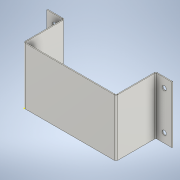
# Autodesk Inventor part: Base Valvula
Saved by Autodesk Inventor 2021 (Build 250183000, 183)
## iProperties
Created: 2021-06-01
Part Number: Base Valvula
Material: Steel AISI 1006 85 HR
Document SubType Name: Chapa
Designer: Admin
Density: 7.872 g/cm^3
Sheet Metal Rule: Default_mm
Appearance: Steel
Flat Pattern Width: 5 cm
Flat Pattern Length: 17.7756 cm
Flat Pattern Area: 88.8782 cm^2
Sheet Metal Width: 50,000 mm
Sheet Metal Length: 177,756 mm
Sheet Metal Area: 8887,816 mm^2
Mass: 52.9731 g
Surface Area: 180.926 cm^2
Volume: 6.72931 cm^3
Author: Admin
Autodesk Inventor part; units mm, degrees
ref_plane "YZ Plane" through (0, 0, 0) normal (1, 0, 0) x (0, 1, 0)
ref_plane "XZ Plane" through (0, 0, 0) normal (0, 1, 0) x (-1, 0, 0)
ref_plane "XY Plane" through (0, 0, 0) normal (0, 0, 1) x (1, 0, 0)
sketch "Boceto1" plane through (0, 0, 0) normal (0, 0, 1) x (1, 0, 0)
  line L0 (0, 0) -> (80, 0)
  line L1 (80, 0) -> (80, 50)
  line L2 (80, 50) -> (0, 50)
  line L3 (0, 50) -> (0, 0)
  dimension "d0" = 80
  dimension "d1" = 50
  measures "d0" distance of L2.end L1.end
  measures "d1" distance of L1.end L0.end
extrude "Placa1" add sketch "Boceto1" along normal blind 0.76
sketch "Boceto2" plane through (80, 50, 0) normal (1, 0, 0) x (0, 1, 0)
  line L0 (-50, 0) -> (0, 0)
  line L1 (0, 0) -> (0, 34.24)
  line L2 (0, 34.24) -> (-50, 34.24)
  line L3 (-50, 34.24) -> (-50, 0)
  constraints: 6 end point, 1 horizontal, 1 perpendicular, 1 vertical
edge flange "Pestaña1" height 35 angle 90 thickness 0.76 bend radius 0.76 thickness toward (1, 0, 0) relief tear relief width 0.76 relief depth 0.38 corner gap 0.76 corner form 0 edges at (80, 25, 0.76) (0, 25, 0.76) wall of the first edge with corners at (80, 0, 0) (80, 50, 0) (80, 50, -34.24) (80, 0, -34.24)
bend "Doblez1"
corner "Esquina1"
sketch "Boceto3" plane through (-0.76, 50, -34.24) normal (0, 0, -1) x (1, 0, 0)
  line L0 (0, -50) -> (0, 0)
  line L1 (0, 0) -> (-14.24, 0)
  line L2 (-14.24, 0) -> (-14.24, -50)
  line L3 (-14.24, -50) -> (0, -50)
  constraints: 6 end point, 1 horizontal, 1 perpendicular, 1 vertical
edge flange "Pestaña2" height 15 angle 90 thickness 0.76 bend radius 0.76 thickness toward (0, 0, -1) relief tear relief width 0.76 relief depth 0.38 corner gap 0.76 corner form 0 edges at (0, 25, -34.24) (80, 25, -34.24) wall of the first edge with corners at (-0.76, 0, -34.24) (-0.76, 50, -34.24) (-15, 50, -34.24) (-15, 0, -34.24)
bend "Doblez2"
corner "Esquina2"
sketch "Boceto4" plane through (-15, 0, -35) normal (0, 0, -1) x (-1, 0, 0)
  circle A0 centre (-6.74, 8) radius 1.95
  circle A1 centre (-6.74, 42) radius 1.95
  point P0 (-15, 0)
  dimension "d23" = 3.9
  dimension "d24" = 3.9
  constraints: 2 centre point, 2 coincident
  measures "d23" diameter of A0
  measures "d24" diameter of A1
extrude "Extrusión1" cut sketch "Boceto4" against normal through all
sketch "Boceto5" plane through (95, 0, -35) normal (0, 0, -1) x (-1, 0, 0)
  circle A0 centre (6.74, 8) radius 1.95
  circle A1 centre (6.74, 42) radius 1.95
  point P0 (95, 0)
  dimension "d27" = 3.9
  dimension "d28" = 3.9
  constraints: 2 centre point, 2 coincident
  measures "d27" diameter of A0
  measures "d28" diameter of A1
extrude "Extrusión2" cut sketch "Boceto5" against normal through all
sketch "Boceto6" plane through (0, 0, 0.76) normal (0, 0, 1) x (1, 0, 0)
  point P0 (0, 0)
equation "\"d24\" = d23"
equation "\"d28\" = d27"
equation "\"d2\" = Grosor"
equation "\"d3\" = Anchura_desahogo_plegado"
equation "\"d4\" = Profundidad_desahogo_plegado"
equation "\"d5\" = Remanente_mínimo"
equation "\"d6\" = Radiodetransición"
equation "\"d9\" = Radio_pliegue"
equation "\"d10\" = Tamaño_destalonado"
equation "\"d11\" = TamañoSeparación"
equation "\"d12\" = Tamaño_de_radio_de_Jacobi"
equation "\"d13\" = Anchura_desahogo_plegado"
equation "\"d14\" = Profundidad_desahogo_plegado"
equation "\"d15\" = Remanente_mínimo"
equation "\"d16\" = Radiodetransición"
equation "\"d19\" = Radio_pliegue"
equation "\"d20\" = Tamaño_destalonado"
equation "\"d21\" = TamañoSeparación"
equation "\"d22\" = Tamaño_de_radio_de_Jacobi"
equation "\"Radio_pliegue\" = Grosor"
equation "\"Anchura_desahogo_plegado\" = Grosor"
equation "\"Profundidad_desahogo_plegado\" = 0.5 * Grosor"
equation "\"Tamaño_destalonado\" = 4 * Grosor"
equation "\"Remanente_mínimo\" = 2 * Grosor"
equation "\"Radiodetransición\" = Radio_pliegue"
equation "\"Tamaño_de_radio_de_Jacobi\" = Radio_pliegue"
equation "\"TamañoSeparación\" = Grosor"
equation "\"Grosor\" = 0.76"
